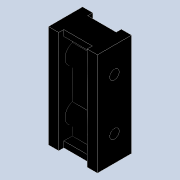
# Autodesk Inventor part: X Axis Belt and V Wheel Plate Spacer
Saved by Autodesk Inventor 2022 (Build 260153000, 153)
## iProperties
Created: 2021-10-13
Part Number: X Axis Belt and V Wheel Plate Spacer
Material: Generic
Document SubType Name: Modeling
Designer: Coy
Density: 1 g/cm^3
Appearance: Anodized - Black
Author: Coy
Autodesk Inventor part; units mm, degrees
ref_plane "YZ Plane" through (0, 0, 0) normal (1, 0, 0) x (0, 1, 0)
ref_plane "XZ Plane" through (0, 0, 0) normal (0, 1, 0) x (-1, 0, 0)
ref_plane "XY Plane" through (0, 0, 0) normal (0, 0, 1) x (1, 0, 0)
sketch "Sketch1" plane through (0, 0, 0) normal (1, 0, 0) x (0, 1, 0)
  line L0 (0, 0) -> (60, 0)
  line L1 (60, 0) -> (60, 20)
  line L2 (60, 20) -> (0, 20)
  line L3 (0, 20) -> (0, 0)
  line L4 (60, 10) -> (0, 10) construction
  line L5 (60, 10) -> (30, 10) construction
  line L6 (30, 10) -> (0, 10) construction
  circle A0 centre (45, 10) radius 2.75
  circle A1 centre (15, 10) radius 2.75
  dimension "d0" = 60
  dimension "d1" = 20
  dimension "d2" = 5.5
  dimension "d3" = 5.5
  constraints: 14 end point, 5 midpoint, 2 centre point, 2 parallel, 1 collinear, 1 horizontal, 1 perpendicular
  measures "d0" distance of L2.end L1.end
  measures "d1" distance of L1.end L0.end
  measures "d2" diameter of A0
  measures "d3" diameter of A1
extrude "Extrusion1" add sketch "Sketch1" against normal blind 6
sketch "Sketch2" plane through (-6, 0, 0) normal (-1, 0, 0) x (0, 0, 1)
  circle A0 centre (10, 45) radius 2.75 projected
  circle A1 centre (10, 15) radius 2.75 projected
  circle A2 centre (10, 45) radius 6.25
  circle A3 centre (10, 15) radius 6.25
  line L0 (20, 60) -> (0, 60) projected
  line L1 (12, 60) -> (12, 0)
  line L2 (8, 60) -> (8, 0)
  line L3 (0, 0) -> (20, 0) projected
  line L4 (0, 60) -> (0, 0) projected
  line L5 (20, 0) -> (20, 60) projected
  line L6 (12, 56.5) -> (17, 56.5)
  line L7 (17, 56.5) -> (17, 60)
  line L8 (8, 56.5) -> (3, 56.5)
  line L9 (3, 56.5) -> (3, 60)
  line L10 (8, 3.5) -> (3, 3.5)
  line L11 (3, 3.5) -> (3, 0)
  line L12 (12, 3.5) -> (17, 3.5)
  line L13 (17, 3.5) -> (17, 0)
  point P0 (12, 39.0786)
  point P1 (12, 50.9214)
  point P2 (8, 50.9214)
  point P3 (8, 39.0786)
  point P4 (8, 20.9214)
  point P5 (8, 9.0786)
  point P6 (12, 9.0786)
  point P7 (12, 20.9214)
  dimension "d6" = 3.5
  dimension "d7" = 8
  dimension "d8" = 8
  dimension "d9" = 3.5
  dimension "d10" = 3.5
  dimension "d11" = 3.5
  dimension "d16" = 3.5
  constraints: 20 end point, 15 point on line, 4 perpendicular, 2 centre point, 2 horizontal, 2 vertical, 1 coincident
  measures "d6" radial gap between concentric circles of A0 A2
  measures "d7" distance between parallel lines of L4 L2
  measures "d8" distance between parallel lines of L5 L1
  measures "d9" distance of L6.end L7.end
  measures "d10" distance of L8.end L9.end
  measures "d11" distance of L12.end L13.end
  measures "d16" radial gap between concentric circles of A1 A3
extrude "Extrusion2" add sketch "Sketch2" along normal blind 16.7 contours A0 L1 A2 | A0 L2 A2 L1 | L1 A2 L2 A0 | A0 L2 A2 | A2 L2 L0 L1 | L1 A3 L2 A2 | L1 L0 L7 L6 | L1 A1 L2 A3 | A3 L1 A1 | L8 L9 L0 L2 | L2 A1 A3 | L2 A1 L1 A3 | A3 L1 L3 L2 | L2 L3 L11 L10 | L12 L13 L3 L1
sketch "Sketch3" plane through (-22.7, 0, 0) normal (-1, 0, 0) x (0, 0, 1)
  circle A0 centre (10, 45) radius 2.75 projected
  circle A1 centre (10, 15) radius 2.75 projected
  line L0 (20, 0) -> (20, 60) projected
  line L1 (17, 0) -> (20, 0) projected
  line L2 (3, 0) -> (17, 0) projected
  line L3 (0, 0) -> (3, 0) projected
  line L4 (0, 60) -> (0, 0) projected
  line L5 (3, 60) -> (0, 60) projected
  line L6 (17, 60) -> (3, 60) projected
  line L7 (20, 60) -> (17, 60) projected
extrude "Extrusion3" add sketch "Sketch3" along normal blind 6
equation "\"d3\" = d2"
equation "\"d16\" = d6"
body "Solid1"
